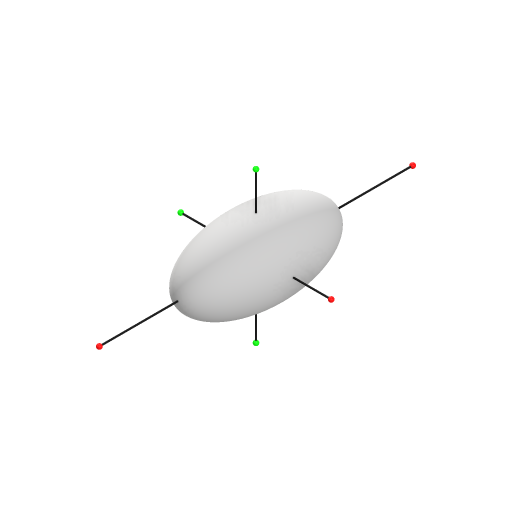
# Autodesk Inventor part: ellipse1
Saved by Autodesk Inventor 2023 (Build 270158000, 158)
## iProperties
Created: 2022-08-07
Part Number: ellipse1
Material: Generic
Document SubType Name: Modeling
Designer: Derm
Density: 1 g/cm^3
Appearance: Default
Author: Derm
Autodesk Inventor part; units mm, degrees
ref_plane "YZ Plane" through (0, 0, 0) normal (1, 0, 0) x (0, 1, 0)
ref_plane "XZ Plane" through (0, 0, 0) normal (0, 1, 0) x (-1, 0, 0)
ref_plane "XY Plane" through (0, 0, 0) normal (0, 0, 1) x (1, 0, 0)
sketch "Sketch1" plane through (0, 0, 0) normal (0, 1, 0) x (-1, 0, 0)
  ellipse E0 centre (0, 0) end of major axis (0, -1250) minor radius 600 (0, -1250) -> (0, 1250) ccw
  line L0 (0, 1250) -> (0, -1250)
  dimension "d0" = 600
  dimension "d1" = 1250
  constraints: 2 end point, 1 coincident, 1 vertical, 4 other
revolve "Revolution1" add sketch "Sketch1" angle 360 about axis through (0, 0, 1250) along (0, 0, -1)
sketch "Sketch2" plane through (0, 0, 0) normal (0, 1, 0) x (-1, 0, 0)
  ellipse E0 centre (0, 0) end of major axis (0, -1250) minor radius 600 (0, -1250) -> (0, 1250) ccw projected
  ellipse E1 centre (0, 0) end of major axis (0, -1239.7967) minor radius 616.7196 (0, -1239.7967) -> (0, 1239.7967) ccw
  line L0 (0, -1239.7967) -> (0, -1250)
  line L1 (0, 1239.7967) -> (0, 1250)
  constraints: 4 end point, 1 collinear, 1 vertical, 5 other
extrude "Extrusion1" [suppressed]
mirror "Mirror1" [suppressed]
sketch "Sketch3" plane through (0, 0, 0) normal (0, 0, 1) x (1, 0, 0)
  circle A0 centre (0, 0) radius 1009.9169
  circle A1 centre (0, 0) radius 989.7967
  constraints: 2 centre point, 2 coincident
extrude "Extrusion2" [suppressed]
sketch "Sketch4" plane through (0, 0, 0) normal (1, 0, 0) x (0, 1, 0)
  line L0 (-5.0643, -10.1808) -> (0, 0) projected
  ellipse E0 centre (0, 0) end of major axis (0, -2003.4356) minor radius 1000.6503
  line L1 (-12.7, -1989.7967) -> (-12.7, -12.7) projected
  ellipse E1 centre (0, 0) end of major axis (0, -1992.4459) minor radius 989.6605
  point P0 (0, -12.7)
  constraints: 2 centre point, 1 coincident, 2 other
extrude "Extrusion3" [suppressed]
sketch "Sketch5" plane through (0, 0, 0) normal (0, 1, 0) x (-1, 0, 0)
  line L0 (0, 0) -> (-1200, 0)
  line L1 (0, 0) -> (1200, 0)
  line L2 (1200, 0) -> (-1200, 0)
  line L3 (-1200, 0) -> (-1200, -12.7)
  line L4 (-1164.079, -12.7) -> (1164.079, -12.7)
  line L5 (1200, -12.7) -> (1200, 0)
  arc A0 (1164.079, -12.7) -> (1238.1, 0) centre (1200, 0) ccw
  arc A1 (-1238.1, 0) -> (-1164.079, -12.7) centre (-1200, 0) ccw
  line L6 (-1200, 0) -> (-1238.1, 0)
  line L7 (1200, 0) -> (1238.1, 0)
  dimension "d9" = 1200
  dimension "d10" = 1200
  dimension "d11" = 12.7
  dimension "d12" = 76.2
  dimension "d13" = 76.2
  constraints: 16 end point, 4 point on circle, 3 horizontal, 2 centre point, 2 coincident, 2 parallel, 2 point on line, 1 perpendicular
  measures "d9" distance of L0.start L1.end
  measures "d10" distance of L0.start L0.end
  measures "d11" distance between parallel lines of L0 L4
  measures "d12" diameter of A0
  measures "d13" diameter of A1
revolve "Revolution2" add sketch "Sketch5" angle 360 about axis through (0, 0, 0) along (-1, 0, 0) separate body
sketch "Sketch6" plane through (0, 0, 0) normal (1, 0, 0) x (0, 1, 0)
  circle A0 centre (0, 0) radius 12.7 projected
  line L0 (0, 0) -> (0, 2500)
  line L1 (0, 0) -> (0, -2500)
  line L2 (0, 2500) -> (12.7, 2500)
  line L3 (12.7, 2464.079) -> (12.7, -2464.079)
  line L4 (12.7, -2500) -> (0, -2500)
  line L5 (0, -2500) -> (0, 2500)
  arc A1 (12.7, 2464.079) -> (0, 2538.1) centre (0, 2500) ccw
  arc A2 (0, -2538.1) -> (12.7, -2464.079) centre (0, -2500) ccw
  line L6 (0, -2500) -> (0, -2538.1)
  line L7 (0, 2500) -> (0, 2538.1)
  dimension "d15" = 2500
  dimension "d16" = 2500
  dimension "d17" = 12.7
  dimension "d18" = 76.2
  dimension "d19" = 76.2
  constraints: 16 end point, 4 point on circle, 2 centre point, 2 coincident, 2 parallel, 2 vertical, 1 horizontal, 1 perpendicular, 1 point on line
  measures "d15" distance of L0.start L0.end
  measures "d16" distance of L0.start L1.end
  measures "d17" distance of L4.start L4.end
  measures "d18" diameter of A1
  measures "d19" diameter of A2
revolve "Revolution3" add sketch "Sketch6" angle 360 about axis through (0, 0, 0) along (0, 0, 1) separate body picked at (2.7788, 7.9413) contours A0 L1 L0 | L3 A2 L6 L1 A0 | A0 L0 L7 A1 L3
sketch "Sketch7" plane through (0, 0, 0) normal (1, 0, 0) x (0, 1, 0)
  line L0 (0, 0) -> (1200, 0)
  line L1 (0, 0) -> (-1200, 0)
  arc A0 (-1238.1, 0) -> (-1164.079, -12.7) centre (-1200, 0) ccw
  arc A1 (1164.079, -12.7) -> (1238.1, 0) centre (1200, 0) ccw
  line L2 (1238.1, 0) -> (-1238.1, 0)
  line L3 (-1238.1, -12.7) -> (-1235.921, -12.7)
  line L4 (-1164.079, -12.7) -> (1164.079, -12.7)
  line L5 (1235.921, -12.7) -> (1238.1, -12.7)
  dimension "d21" = 1200
  dimension "d22" = 1200
  dimension "d23" = 76.2
  dimension "d24" = 76.2
  constraints: 12 end point, 6 point on circle, 3 horizontal, 3 parallel, 2 centre point, 2 coincident
  measures "d21" distance of L0.start L1.end
  measures "d22" distance of L0.start L0.end
  measures "d23" diameter of A0
  measures "d24" diameter of A1
revolve "Revolution4" add sketch "Sketch7" angle 360 about axis through (0, 1238.1, 0) along (0, -1, 0) separate body
body "Solid1"
body "Solid2"
body "Solid3"
body "Solid4"
